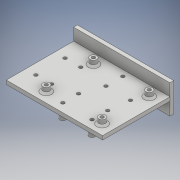
# Autodesk Inventor part: Eletronica - Raspberry
Saved by Autodesk Inventor 2017 (Build 210142000, 142)
## iProperties
Created: 2020-10-24
Part Number: Eletronica - Raspberry
Material: Generic
Document SubType Name: Modeling
Designer: ale
Density: 1 g/cm^3
Appearance: Default
Author: ale
Autodesk Inventor part; units mm, degrees
ref_plane "YZ Plane" through (0, 0, 0) normal (1, 0, 0) x (0, 1, 0)
ref_plane "XZ Plane" through (0, 0, 0) normal (0, 1, 0) x (-1, 0, 0)
ref_plane "XY Plane" through (0, 0, 0) normal (0, 0, 1) x (1, 0, 0)
sketch "Sketch1" plane through (0, 0, 0) normal (0, 0, 1) x (1, 0, 0)
  line L0 (-42.5, 28) -> (42.5, 28)
  line L1 (42.5, 28) -> (42.5, -28)
  line L2 (42.5, -28) -> (-42.5, -28)
  line L3 (-42.5, -28) -> (-42.5, 28)
  line L4 (-42.5, 28) -> (42.5, -28) construction
  line L5 (42.5, 28) -> (-42.5, -28) construction
  line L6 (-50, 35) -> (50, 35)
  line L7 (50, 35) -> (50, -35)
  line L8 (50, -35) -> (-50, -35)
  line L9 (-50, -35) -> (-50, 35)
  line L10 (-50, 35) -> (50, -35) construction
  line L11 (50, 35) -> (-50, -35) construction
  circle A0 centre (39, -24.5) radius 3.5
  circle A1 centre (39, 24.5) radius 3.5
  circle A2 centre (-19, 24.5) radius 3.5
  circle A3 centre (-19, -24.5) radius 3.5
  point P0 (0, 0)
  dimension "d0" = 85
  dimension "d1" = 56
  dimension "d2" = 100
  dimension "d3" = 70
  dimension "d4" = 7
  dimension "d5" = 7
  dimension "d6" = 3.5
  dimension "d7" = 3.5
  dimension "d8" = 3.5
  dimension "d9" = 3.5
  dimension "d10" = 7
  dimension "d11" = 7
  dimension "d12" = 58
  dimension "d13" = 58
  dimension "d14" = 3.5
  dimension "d15" = 3.5
  constraints: 24 end point, 4 centre point, 4 midpoint, 4 parallel, 2 horizontal, 2 perpendicular
  measures "d0" distance of L1.end L2.end
  measures "d1" distance of L0.end L1.end
  measures "d2" distance of L7.end L8.end
  measures "d3" distance of L6.end L7.end
  measures "d4" diameter of A0
  measures "d5" diameter of A1
  measures "d6" distance from line of A1.centre L1
  measures "d7" distance from line of A1.centre L0
  measures "d8" distance from line of A0.centre L1
  measures "d9" distance from line of A0.centre L2
  measures "d10" diameter of A2
  measures "d11" diameter of A3
  measures "d12" distance of A1.centre A2.centre
  measures "d13" distance of A3.centre A0.centre
  measures "d14" distance from line of A2.centre L0
  measures "d15" distance from line of A3.centre L2
extrude "Extrusion1" add sketch "Sketch1" along normal blind 4 contours L0 A1 L1 A0 L2 L3 | L0 L1 A1 | A0 L1 L2 | L6 L7 L8 L9
sketch "Sketch2" plane through (0, 0, 0) normal (0, 0, -1) x (-1, 0, 0)
  circle A0 centre (19, 24.5) radius 3.5 projected
  circle A1 centre (19, 24.5) radius 3.5
  circle A2 centre (19, 24.5) radius 1.75
  circle A3 centre (-39, 24.5) radius 3.5 projected
  circle A4 centre (-39, 24.5) radius 3.5
  circle A5 centre (-39, 24.5) radius 1.75
  circle A6 centre (-39, -24.5) radius 3.5 projected
  circle A7 centre (-39, -24.5) radius 3.5
  circle A8 centre (-39, -24.5) radius 1.75
  circle A9 centre (19, -24.5) radius 3.5 projected
  circle A10 centre (19, -24.5) radius 3.5
  circle A11 centre (19, -24.5) radius 1.75
  point P0 (0, 0)
  dimension "d18" = 3.5
  dimension "d19" = 3.5
  dimension "d20" = 3.5
  dimension "d21" = 3.5
  constraints: 8 centre point, 8 coincident
  measures "d18" diameter of A2
  measures "d19" diameter of A5
  measures "d20" diameter of A8
  measures "d21" diameter of A11
extrude "Extrusion2" add sketch "Sketch2" against normal blind 10
sketch "Sketch3" plane through (0, 0, 0) normal (0, 0, -1) x (-1, 0, 0)
  line L0 (-38.5, 31.075) -> (-1.5, 31.075)
  line L1 (-1.5, 31.075) -> (-1.5, 8.925)
  line L2 (-1.5, 8.925) -> (-38.5, 8.925)
  line L3 (-38.5, 8.925) -> (-38.5, 31.075)
  line L4 (-38.5, 31.075) -> (-1.5, 8.925) construction
  line L5 (-1.5, 31.075) -> (-38.5, 8.925) construction
  line L6 (-50, 35) -> (-50, -35) projected
  line L7 (50, 35) -> (-50, 35) projected
  line L8 (-32.75, 28.75) -> (-7.25, 28.75)
  line L9 (-7.25, 28.75) -> (-7.25, 11.25)
  line L10 (-7.25, 11.25) -> (-32.75, 11.25)
  line L11 (-32.75, 11.25) -> (-32.75, 28.75)
  line L12 (-32.75, 28.75) -> (-7.25, 11.25) construction
  line L13 (-7.25, 28.75) -> (-32.75, 11.25) construction
  circle A0 centre (-32.75, 28.75) radius 3
  circle A1 centre (-7.25, 28.75) radius 3
  circle A2 centre (-7.25, 11.25) radius 3
  circle A3 centre (-32.75, 11.25) radius 3
  circle A4 centre (-32.75, 11.25) radius 1.75
  circle A5 centre (-32.75, 28.75) radius 1.75
  circle A6 centre (-7.25, 28.75) radius 1.75
  circle A7 centre (-7.25, 11.25) radius 1.75
  point P0 (0, 0)
  point P1 (-20, 20)
  dimension "d24" = 37
  dimension "d25" = 22.15
  dimension "d26" = 30
  dimension "d28" = 15
  dimension "d29" = 25.5
  dimension "d30" = 17.5
  dimension "d31" = 6
  dimension "d32" = 6
  dimension "d33" = 6
  dimension "d34" = 6
  dimension "d35" = 3.5
  dimension "d36" = 3.5
  dimension "d37" = 3.5
  dimension "d38" = 3.5
  constraints: 24 end point, 8 centre point, 8 coincident, 4 midpoint, 4 parallel, 2 horizontal, 2 perpendicular
  measures "d24" distance of L1.end L2.end
  measures "d25" distance of L0.end L1.end
  measures "d26" distance from line of L6 point (-20, 20)
  measures "d28" distance from line of L7 point (-20, 20)
  measures "d29" distance of L9.end L10.end
  measures "d30" distance of L8.end L9.end
  measures "d31" diameter of A0
  measures "d32" diameter of A1
  measures "d33" diameter of A2
  measures "d34" diameter of A3
  measures "d35" diameter of A4
  measures "d36" diameter of A5
  measures "d37" diameter of A6
  measures "d38" diameter of A7
extrude "Extrusion3" add sketch "Sketch3" along normal blind 10 contours A0 L0 | L0 A0 L8 A5 L11 | L11 A5 L8 A0 | A3 L11 A4 L10 L2 | L2 A3 | A1 L0 | L0 A1 L9 A6 L8 | A3 L10 A4 L11 | L8 A6 L9 A1 | A2 L10 A7 L9 L2 | L2 A2 | A2 L9 A7 L10
sketch "Sketch5" plane through (0, 0, 0) normal (0, 0, -1) x (-1, 0, 0)
  line L0 (-36.5, -7.5) -> (6.5, -7.5)
  line L1 (6.5, -7.5) -> (6.5, -28.5)
  line L2 (6.5, -28.5) -> (-36.5, -28.5)
  line L3 (-36.5, -28.5) -> (-36.5, -7.5)
  line L4 (-36.5, -7.5) -> (6.5, -28.5) construction
  line L5 (6.5, -7.5) -> (-36.5, -28.5) construction
  line L6 (-50, -35) -> (50, -35) projected
  line L7 (-50, 35) -> (-50, -35) projected
  line L8 (-30.15, -9.85) -> (0.15, -9.85)
  line L9 (0.15, -9.85) -> (0.15, -26.15)
  line L10 (0.15, -26.15) -> (-30.15, -26.15)
  line L11 (-30.15, -26.15) -> (-30.15, -9.85)
  line L12 (-30.15, -9.85) -> (0.15, -26.15) construction
  line L13 (0.15, -9.85) -> (-30.15, -26.15) construction
  circle A0 centre (0.15, -9.85) radius 3
  circle A1 centre (-30.15, -9.85) radius 3
  circle A2 centre (-30.15, -26.15) radius 3
  circle A3 centre (0.15, -26.15) radius 3
  line L14 (20.5, -21.5) -> (20.5, 21.5)
  line L15 (20.5, 21.5) -> (41.5, 21.5)
  line L16 (41.5, 21.5) -> (41.5, -21.5)
  line L17 (41.5, -21.5) -> (20.5, -21.5)
  line L18 (20.5, -21.5) -> (41.5, 21.5) construction
  line L19 (20.5, 21.5) -> (41.5, -21.5) construction
  line L20 (22.85, -15.15) -> (22.85, 15.15)
  line L21 (22.85, 15.15) -> (39.15, 15.15)
  line L22 (39.15, 15.15) -> (39.15, -15.15)
  line L23 (39.15, -15.15) -> (22.85, -15.15)
  line L24 (22.85, -15.15) -> (39.15, 15.15) construction
  line L25 (22.85, 15.15) -> (39.15, -15.15) construction
  circle A4 centre (22.85, 15.15) radius 3
  circle A5 centre (22.85, -15.15) radius 3
  circle A6 centre (39.15, -15.15) radius 3
  circle A7 centre (39.15, 15.15) radius 3
  line L26 (50, -35) -> (50, 35) projected
  point P0 (0, 0)
  point P1 (-15, -18)
  point P2 (31, 0)
  dimension "d49" = 43
  dimension "d50" = 21
  dimension "d51" = 17
  dimension "d52" = 35
  dimension "d53" = 30.3
  dimension "d54" = 16.3
  dimension "d55" = 6
  dimension "d56" = 6
  dimension "d57" = 6
  dimension "d58" = 6
  dimension "d59" = 43
  dimension "d60" = 21
  dimension "d61" = 30.3
  dimension "d62" = 16.3
  dimension "d63" = 6
  dimension "d64" = 6
  dimension "d65" = 6
  dimension "d66" = 6
  dimension "d67" = 35
  dimension "d68" = 19
  constraints: 48 end point, 8 centre point, 8 coincident, 8 midpoint, 8 parallel, 4 perpendicular, 2 horizontal
  measures "d49" distance of L1.end L2.end
  measures "d50" distance of L0.end L1.end
  measures "d51" distance from line of L6 point (-15, -18)
  measures "d52" distance from line of L7 point (-15, -18)
  measures "d53" distance of L9.end L10.end
  measures "d54" distance of L8.end L9.end
  measures "d55" diameter of A0
  measures "d56" diameter of A1
  measures "d57" diameter of A2
  measures "d58" diameter of A3
  measures "d59" distance of L18.end L17.start
  measures "d60" distance of L14.end L18.end
  measures "d61" distance of L22.start L23.start
  measures "d62" distance of L20.end L22.start
  measures "d63" diameter of A4
  measures "d64" diameter of A5
  measures "d65" diameter of A6
  measures "d66" diameter of A7
  measures "d67" distance from line of point (31, 0) L6
  measures "d68" distance from line of L26 point (31, 0)
extrude "Extrusion4" add sketch "Sketch5" along normal blind 10 contours A1 L0 | L0 A1 L8 L11 | L11 L8 A1 | A2 L11 L10 L2 | L2 A2 | A0 L0 | L0 A0 L9 L8 | A2 L10 L11 | L8 L9 A0 | A3 L10 L9 L2 | L2 A3 | A3 L9 L10 | A5 L14 | L14 A5 L20 L23 | L23 L20 A5 | A6 L23 L22 L16 | L16 A6 | A4 L14 | L14 A4 L21 L20 | A6 L22 L23 | L20 L21 A4 | A7 L22 L21 L16 | L16 A7 | A7 L21 L22
sketch "Sketch6" plane through (32.75, 28.75, -10) normal (0, 0, -1) x (-1, 0, 0)
  circle A0 centre (0, 0) radius 1.75 projected
  circle A1 centre (25.5, 0) radius 1.75 projected
  circle A2 centre (25.5, -17.5) radius 1.75 projected
  circle A3 centre (0, -17.5) radius 1.75 projected
  circle A4 centre (2.6, -38.6) radius 3 projected
  circle A5 centre (2.6, -54.9) radius 3 projected
  circle A6 centre (32.9, -54.9) radius 3 projected
  circle A7 centre (32.9, -38.6) radius 3 projected
  circle A8 centre (55.6, -43.9) radius 3 projected
  circle A9 centre (55.6, -13.6) radius 3 projected
  circle A10 centre (71.9, -13.6) radius 3 projected
  circle A11 centre (71.9, -43.9) radius 3 projected
  point P0 (32.75, -28.75)
  constraints: 12 coincident
hole "Hole2" at (32.75, 28.75, -10) at (7.25, 28.75, -10) at (7.25, 11.25, -10) at (32.75, 11.25, -10) at (30.15, -9.85, -10) at (30.15, -26.15, -10) at (-0.15, -26.15, -10) at (-0.15, -9.85, -10) at (-22.85, -15.15, -10) at (-22.85, 15.15, -10) at (-39.15, 15.15, -10) at (-39.15, -15.15, -10) at (32.75, 28.75, -10) at (7.25, 28.75, -10) at (7.25, 11.25, -10) at (32.75, 11.25, -10) at (30.15, -9.85, -10) at (30.15, -26.15, -10) at (-0.15, -9.85, -10) at (-0.15, -26.15, -10) at (-22.85, -15.15, -10) at (-39.15, -15.15, -10) at (-39.15, 15.15, -10) at (-22.85, 15.15, -10) direction (0, 0, 1) diameter 3.5 end through all
chamfer "Chamfer1" distance 2 angle 45 15 edges at (35.75, 28.75, 0) (35.75, 11.25, 0) (10.25, 28.75, 0) (10.25, 11.25, 0) (-19.85, 15.15, 0) (2.85, -9.85, 0) (-19.85, -15.15, 0) (2.85, -26.15, 0) (33.15, -26.15, 0) (-36.15, 15.15, 0) (-36.15, -15.15, 0) (-15.5, -24.5, 4) (-15.5, 24.5, 4) (42.5, 24.5, 4) (42.5, -24.5, 4)
sketch "Sketch7" plane through (-50, 35, 0) normal (0, 1, 0) x (1, 0, 0)
  line L0 (-0.15, 13.5) -> (99.85, 13.5)
  line L1 (99.85, 13.5) -> (99.85, -16.5)
  line L2 (99.85, -16.5) -> (-0.15, -16.5)
  line L3 (-0.15, -16.5) -> (-0.15, 13.5)
  line L4 (-0.15, 13.5) -> (99.85, -16.5) construction
  line L5 (99.85, 13.5) -> (-0.15, -16.5) construction
  line L6 (0, 0) -> (100, 0) projected
  point P0 (50, 0)
  point P1 (49.85, -1.5)
  dimension "d81" = 100
  dimension "d82" = 30
  dimension "d83" = 1.5
  constraints: 12 end point, 2 midpoint, 2 parallel, 1 horizontal, 1 perpendicular
  measures "d81" distance of L1.end L2.end
  measures "d82" distance of L0.end L1.end
  measures "d83" distance from line of L6 point (49.85, -1.5)
extrude "Extrusion5" add sketch "Sketch7" along normal blind 4
sketch "Sketch8" plane through (-50, 35, 0) normal (0, -1, 0) x (1, 0, 0)
  line L0 (99.85, 16.5) -> (-0.15, 16.5) projected
  line L1 (99.85, 4) -> (99.85, 16.5) projected
  point P0 (50, 0)
  point P1 (66.5167, -6)
  point P2 (33.1833, -6)
  dimension "d86" = 22.5
  dimension "d87" = 22.5
  dimension "d88" = 33.3333
  dimension "d89" = 66.6667
  measures "d86" distance from line of L0 point (33.183, -6)
  measures "d87" distance from line of L0 point (66.517, -6)
  measures "d88" distance from line of L1 point (66.517, -6)
  measures "d89" distance from line of L1 point (33.183, -6)
hole "Hole3" at (16.5167, 35, -6) at (-16.8167, 35, -6) direction (0, 1, 0) diameter 5 end through all
equation "\"d4\" = d10"
equation "\"d5\" = d10"
equation "\"d11\" = d10"
equation "\"d13\" = d12"
body "Solid1"
